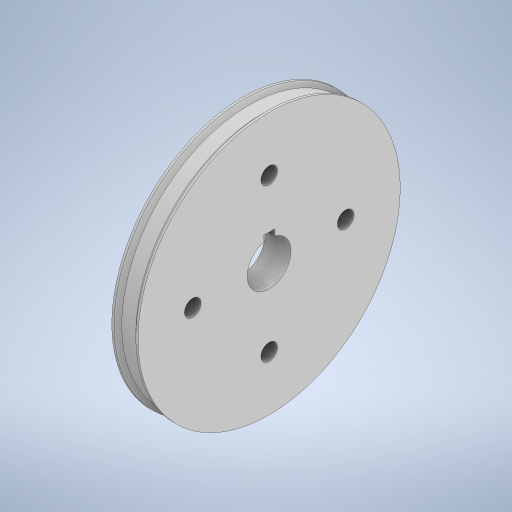
# Autodesk Inventor part: Polea-1021920
Saved by Autodesk Inventor 2024 (Build 280153000, 153)
## iProperties
Created: 2024-02-06
Part Number: Polea-1021920
Material: Generic
Document SubType Name: Modeling
Designer: JavierJ
Density: 1 g/cm^3
Appearance: Default
Author: JavierJ
Autodesk Inventor part; units mm, degrees
ref_plane "YZ Plane" through (0, 0, 0) normal (1, 0, 0) x (0, 1, 0)
ref_plane "XZ Plane" through (0, 0, 0) normal (0, 1, 0) x (-1, 0, 0)
ref_plane "XY Plane" through (0, 0, 0) normal (0, 0, 1) x (1, 0, 0)
sketch "Sketch1" plane through (0, 0, 0) normal (0, 0, 1) x (1, 0, 0)
  line L0 (0, 0) -> (100, 0)
  line L1 (100, 0) -> (100, 500)
  line L2 (0, 500) -> (0, 0)
  line L3 (0, 500) -> (17.6777, 482.3223)
  line L4 (100, 500) -> (82.3223, 482.3223)
  line L5 (17.6777, 482.3223) -> (82.3223, 482.3223)
  line L6 (50, -100) -> (-150, -100)
  constraints: 14 end point, 3 horizontal, 1 parallel, 1 perpendicular
revolve "Revolution1" add sketch "Sketch1" angle 360 about axis through (50, -100, 0) along (-1, 0, 0)
sketch "Sketch2" plane through (100, -100, 0) normal (1, 0, 0) x (0, 0, -1)
  circle A0 centre (0, 0) radius 600 projected
  circle A1 centre (0, 350) radius 37.5
  circle A2 centre (0, 0) radius 100 projected
  circle A3 centre (-350, 0) radius 37.5
  circle A4 centre (0, -350) radius 37.5
  circle A5 centre (350, 0) radius 37.5
  point P0 (0, 100)
  dimension "d8" = 360
  constraints: 4 centre point, 1 vertical alignment, 9 other
extrude "Extrusion1" cut sketch "Sketch2" against normal blind 100 contours A1 | A3 | A4 | A5
thicken "Thicken1" operation add thickness 10 both sides no extend neighbours no toward (1, 0, 0) faces at (100, -364.9419, 262.9039)
thicken "Thicken2" operation add thickness 10 both sides no extend neighbours no toward (-1, 0, 0) faces at (0, -364.9419, 262.9039)
sketch "Sketch3" plane through (110, -100, 0) normal (1, 0, 0) x (0, 0, -1)
  line L0 (-25, 125) -> (25, 125)
  line L1 (25, 125) -> (25, 96.8246)
  line L2 (-25, 96.8246) -> (-25, 125)
  line L3 (-25, 125) -> (0, 100) construction
  line L4 (25, 125) -> (0, 100) construction
  arc A0 (25, 96.8246) -> (-25, 96.8246) centre (0, 0) ccw
  point P0 (0, 100)
  constraints: 10 end point, 3 point on circle, 2 point on line, 1 centre point, 1 horizontal, 1 parallel, 1 perpendicular
extrude "Extrusion2" cut sketch "Sketch3" against normal blind 120
body "Solid1"
